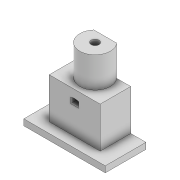
# Autodesk Inventor part: Feather_0_template
Saved by Autodesk Inventor 2022 (Build 260153000, 153)
## iProperties
Created: 2022-08-10
Part Number: Feather_0_template
Material: Generic
Document SubType Name: Modeling
Designer: dell
Density: 1 g/cm^3
Appearance: Default
Author: dell
Autodesk Inventor part; units mm, degrees
ref_plane "YZ Plane" through (0, 0, 0) normal (1, 0, 0) x (0, 1, 0)
ref_plane "XZ Plane" through (0, 0, 0) normal (0, 1, 0) x (-1, 0, 0)
ref_plane "XY Plane" through (0, 0, 0) normal (0, 0, 1) x (1, 0, 0)
sketch "Sketch1" plane through (0, 0, 0) normal (0, 0, 1) x (1, 0, 0)
  circle A0 centre (0, 0) radius 6.1
  line L0 (-12.5, -10) -> (12.5, -10)
  line L1 (12.5, -10) -> (12.5, 10)
  line L2 (12.5, 10) -> (-12.5, 10)
  line L3 (-12.5, 10) -> (-12.5, -10)
  line L4 (-12.5, -10) -> (12.5, 10) construction
  line L5 (12.5, -10) -> (-12.5, 10) construction
  dimension "d0" = 12.2
  dimension "d1" = 25
  dimension "d2" = 20
  constraints: 12 end point, 2 midpoint, 2 parallel, 1 centre point, 1 coincident, 1 horizontal, 1 perpendicular
  measures "d0" diameter of A0
  measures "d1" distance between parallel lines of L3 L1
  measures "d2" distance between parallel lines of L2 L0
extrude "Extrusion1" add sketch "Sketch1" along normal blind 20
sketch "Sketch2" plane through (-12.5, 10, 0) normal (0, 1, 0) x (1, 0, 0)
  line L0 (0, 0) -> (0, -20) construction
  line L1 (25, -20) -> (0, -20) construction
  line L2 (0, 0) -> (25, -20) construction
  line L3 (0, -20) -> (25, 0) construction
  circle A0 centre (12.5, -10) radius 1.95
  point P0 (12.5, 0)
  dimension "d5" = 3.9
  constraints: 4 end point, 1 centre point, 1 midpoint
  measures "d5" diameter of A0
extrude "Extrusion2" cut sketch "Sketch2" against normal blind 100
sketch "Sketch3" plane through (-12.5, 10, 0) normal (0, 1, 0) x (1, 0, 0)
  circle A0 centre (12.5, -10) radius 1.95 projected
  line L0 (25, 0) -> (0, 0) projected
  line L1 (0, 0) -> (0, -20) projected
  line L2 (25, -20) -> (0, -20) projected
  line L3 (25, 0) -> (25, -20) projected
  circle A1 centre (12.5, -10) radius 7.5
  point P0 (12.5, 0)
  dimension "d8" = 15
  constraints: 1 centre point, 1 coincident
  measures "d8" diameter of A1
extrude "Extrusion3" add sketch "Sketch3" along normal blind 15 contours A1
sketch "Sketch4" plane through (-12.5, -10, 0) normal (0, -1, 0) x (1, 0, 0)
  line L0 (32.5, 25) -> (-7.5, 25)
  line L1 (-7.5, 25) -> (-7.5, -5)
  line L2 (-7.5, -5) -> (32.5, -5)
  line L3 (32.5, -5) -> (32.5, 25)
  circle A0 centre (12.5, 10) radius 1.95 projected
  line L4 (32.5, 25) -> (-7.5, -5) construction
  line L5 (-7.5, 25) -> (32.5, -5) construction
  point P0 (12.5, 0)
  dimension "d11" = 30
  dimension "d12" = 40
  constraints: 12 end point, 2 midpoint, 2 parallel, 1 horizontal, 1 perpendicular
  measures "d11" distance of L0.end L1.end
  measures "d12" distance of L1.end L2.end
extrude "Extrusion4" add sketch "Sketch4" along normal blind 3
sketch "Sketch6" plane through (20, -10, -5) normal (0, 0, -1) x (-1, 0, 0)
  line L0 (-13.3468, 43.0165) -> (63.7046, 43.0165)
  line L1 (63.7046, 43.0165) -> (63.7046, -16.6019)
  line L2 (63.7046, -16.6019) -> (-13.3468, -16.6019)
  line L3 (-13.3468, -16.6019) -> (-13.3468, 43.0165)
  point P0 (20, 10)
  constraints: 8 end point, 2 parallel, 1 horizontal, 1 perpendicular
extrude "Extrusion6" cut sketch "Sketch6" against normal blind 10
sketch "Sketch8" plane through (-12.5, 25, 0) normal (0, 1, 0) x (1, 0, 0)
  circle A0 centre (12.5, -10) radius 1.95 projected
  point P0 (12.5, 0)
extrude "Extrusion8" cut sketch "Sketch8" against normal blind 100
sketch "Sketch9" plane through (0, 0, 20) normal (0, 0, 1) x (1, 0, 0)
  line L0 (-2, 5.7628) -> (-2, 3)
  line L1 (-2, 3) -> (2, 3)
  line L2 (2, 3) -> (2, 5.7628)
  circle A0 centre (0, 0) radius 6.1 projected
  line L3 (12.5, -10) -> (12.5, 10) projected
  line L4 (12.5, 10) -> (-12.5, 10) projected
  line L5 (-12.5, 10) -> (-12.5, -10) projected
  line L6 (-12.5, -10) -> (12.5, -10) projected
  circle A1 centre (0, 0) radius 6.1 projected
  dimension "d28" = 2
  dimension "d29" = 2
  dimension "d30" = 3
  constraints: 6 end point, 2 perpendicular, 2 point on circle, 1 vertical
  measures "d28" distance from line of point (0, 0) L2
  measures "d29" distance from line of point (0, 0) L0
  measures "d30" distance from line of point (0, 0) L1
extrude "Extrusion9" add sketch "Sketch9" against normal blind 5 contours L0 L1 L2 A0 picked at (0.2259, -0.0207)
sketch "Sketch10" plane through (0, 0, 15) normal (0, 0, -1) x (-1, 0, 0)
  circle A0 centre (0, 0) radius 4.9
  dimension "d33" = 9.8
  constraints: 1 centre point, 1 coincident
  measures "d33" diameter of A0
extrude "Extrusion10" add sketch "Sketch10" along normal blind 15
sketch "Sketch11" plane through (-12.5, 25, 0) normal (0, 1, 0) x (1, 0, 0)
  circle A0 centre (12.5, -10) radius 1.95 projected
  point P0 (12.5, 0)
extrude "Extrusion11" cut sketch "Sketch11" against normal blind 100
body "Solid1"
